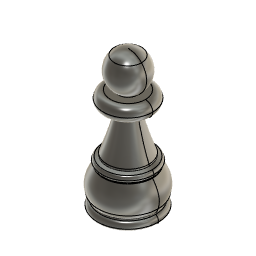
Pawn Chess -HW 3 v1 (Autodesk Fusion 360 design; units mm, degrees)
Autodesk Fusion 360 part; units mm, degrees
sketch "Sketch1" plane through (0, 0, 0) normal (0, 1, 0) x (1, 0, 0)
  line L0 (72.5944, -8.4387) -> (65.6335, -8.4387)
  spline S0 degree 3 poles (65.6335, -8.4387) (65.4687, -8.5077) (65.3491, -8.631) (65.3922, -8.8427) knots 0 0 0 0 1 1 1 1
  spline S1 degree 3 poles (65.3922, -8.8427) (65.4356, -9.0559) (65.5427, -9.1507) (65.6798, -9.194) knots 0 0 0 0 1 1 1 1
  line L1 (65.6798, -9.194) -> (72.4997, -9.194)
  spline S2 degree 3 poles (72.4997, -9.194) (72.6653, -9.1226) (72.7505, -8.9684) (72.7553, -8.7413) knots 0 0 0 0 1 1 1 1
  spline S3 degree 3 poles (72.7553, -8.7413) (72.759, -8.5659) (72.6936, -8.4802) (72.5944, -8.4387) knots 0 0 0 0 1 1 1 1
  line L2 (72.8397, -4.2522) -> (65.3954, -4.2522)
  spline S4 degree 3 poles (65.3954, -4.2522) (65.1932, -4.3686) (65.0932, -4.6054) (64.9953, -4.8506) knots 0 0 0 0 1 1 1 1
  spline S5 degree 3 poles (64.9953, -4.8506) (64.6749, -5.6502) (64.7802, -6.435) (65.0945, -7.2004) knots 0 0 0 0 1 1 1 1
  spline S6 degree 3 poles (65.0945, -7.2004) (65.2549, -7.5909) (65.4192, -7.9897) (65.7398, -8.2884) knots 0 0 0 0 1 1 1 1
  line L3 (65.7398, -8.2884) -> (72.5039, -8.2884)
  spline S7 degree 3 poles (72.5039, -8.2884) (72.5275, -8.2749) (72.5494, -8.2572) (72.569, -8.2312) knots 0 0 0 0 1 1 1 1
  spline S8 degree 3 poles (72.569, -8.2312) (73.3077, -7.248) (73.7827, -6.2021) (73.3307, -4.943) knots 0 0 0 0 1 1 1 1
  spline S9 degree 3 poles (73.3307, -4.943) (73.1731, -4.5035) (73.0804, -4.3233) (72.8397, -4.2522) knots 0 0 0 0 1 1 1 1
  line L4 (65.3755, -4.1021) -> (72.981, -4.1021)
  spline S10 degree 3 poles (72.981, -4.1021) (73.2561, -4.0127) (73.4151, -3.7381) (73.3826, -3.3936) knots 0 0 0 0 1 1 1 1
  spline S11 degree 3 poles (73.3826, -3.3936) (73.3461, -3.0062) (73.0315, -3.1843) (72.8611, -3.1822) knots 0 0 0 0 1 1 1 1
  spline S12 degree 3 poles (72.8611, -3.1822) (71.3313, -3.1645) (69.8012, -3.1737) (68.2714, -3.1753) knots 0 0 0 0 1 1 1 1
  spline S13 degree 3 poles (68.2714, -3.1753) (67.2456, -3.1758) (66.2193, -3.184) (65.1935, -3.1753) knots 0 0 0 0 1 1 1 1
  spline S14 degree 3 poles (65.1935, -3.1753) (64.9379, -3.1727) (64.8837, -3.26) (64.9358, -3.4978) knots 0 0 0 0 1 1 1 1
  spline S15 degree 3 poles (64.9358, -3.4978) (65.0101, -3.8389) (65.1136, -4.0093) (65.3755, -4.1021) knots 0 0 0 0 1 1 1 1
  spline S16 degree 3 poles (67.7795, -14.6889) (67.8422, -14.9569) (67.8525, -15.0773) (67.7568, -15.1308) knots 0 0 0 0 1 1 1 1
  line L5 (67.7568, -15.1308) -> (66.7768, -15.1308)
  spline S17 degree 3 poles (66.7768, -15.1308) (66.219, -15.1308) (65.7668, -15.5829) (65.7668, -16.1409) knots 0 0 0 0 1 1 1 1
  spline S18 degree 3 poles (65.7668, -16.1409) (65.7668, -16.6987) (66.219, -17.1511) (66.7768, -17.1511) knots 0 0 0 0 1 1 1 1
  line L6 (66.7768, -17.1511) -> (67.7938, -17.1511)
  spline S19 degree 3 poles (67.7938, -17.1511) (67.8033, -17.1543) (67.8126, -17.1569) (67.8219, -17.1604) knots 0 0 0 0 1 1 1 1
  spline S20 degree 3 poles (67.8219, -17.1604) (66.1568, -18.3497) (66.3346, -20.2592) (67.299, -21.2874) knots 0 0 0 0 1 1 1 1
  spline S21 degree 3 poles (67.299, -21.2874) (68.2301, -22.2798) (69.9827, -22.3899) (71.0477, -21.2707) knots 0 0 0 0 1 1 1 1
  spline S22 degree 3 poles (71.0477, -21.2707) (71.8814, -20.3947) (72.2721, -18.5463) (70.5103, -17.1511) knots 0 0 0 0 1 1 1 1
  line L7 (70.5103, -17.1511) -> (71.5856, -17.1511)
  spline S23 degree 3 poles (71.5856, -17.1511) (72.1433, -17.1511) (72.5957, -16.6987) (72.5957, -16.1409) knots 0 0 0 0 1 1 1 1
  spline S24 degree 3 poles (72.5957, -16.1409) (72.5957, -15.5829) (72.1433, -15.1308) (71.5856, -15.1308) knots 0 0 0 0 1 1 1 1
  line L8 (71.5856, -15.1308) -> (70.6344, -15.1308)
  spline S25 degree 3 poles (70.6344, -15.1308) (70.4441, -15.0678) (70.4735, -14.9019) (70.5854, -14.4611) knots 0 0 0 0 1 1 1 1
  spline S26 degree 3 poles (70.5854, -14.4611) (70.9987, -12.8305) (71.4265, -11.2041) (72.0682, -9.6452) knots 0 0 0 0 1 1 1 1
  spline S27 degree 3 poles (72.0682, -9.6452) (72.1309, -9.4933) (72.1171, -9.4266) (72.0494, -9.3906) knots 0 0 0 0 1 1 1 1
  line L9 (72.0494, -9.3906) -> (66.0849, -9.3906)
  spline S28 degree 3 poles (66.0849, -9.3906) (65.9841, -9.4652) (66.0304, -9.5613) (66.1489, -9.8372) knots 0 0 0 0 1 1 1 1
  spline S29 degree 3 poles (66.1489, -9.8372) (66.8254, -11.4099) (67.3874, -13.0212) (67.7795, -14.6889) knots 0 0 0 0 1 1 1 1
  line L10 (69.1782, -3.1737) -> (69.1782, -22.0713)
  constraint coincident S12 L10.start
  constraint coincident S21 L10.end
  constraint perpendicular L9 L10
revolve "Revolve1" add sketch "Sketch1" angle 360 about axis through (69.1782, 0, 3.1737) along (0, 0, 1) contours L0 L1 S2 S3 L10 | L2 L3 S7 S8 S9 L10 | L4 S10 S11 S12 L10 | S21 S22 L7 S23 S24 L8 S25 S26 S27 L9 L10 makes body 1 at (68.1456, -0.1331, 8.4387) makes body 2 at (65.9271, 2.2166, 7.387) makes body 3 at (71.4789, -0.2302, 11.2242) makes body 4 at (68.6008, -0.6788, 4.1021)
loft "Loft1" add section 1 face at (69.9805, -0.0503, 9.3906) section 2 face at (68.754, 0.2624, 9.194) on bodies 1 3 bodies 3 1
loft "Loft2" add section 1 face at (68.1057, 0.0267, 8.4387) section 2 face at (68.279, 0.5259, 8.2884) on bodies 2 3 bodies 3 2
loft "Loft3" add section 1 face at (70.1414, -0.7496, 4.2522) section 2 face at (67.9727, -0.3917, 4.1021) on bodies 3 4 bodies 3 4
copy_body "Body->Comp1" bodies 3 removing the originals makes body 5 in component "Component"
component "Component" placed x (1, 0, 0) y (0, 1, 0) z (0, 0, 1) at (0, 0, 0)
